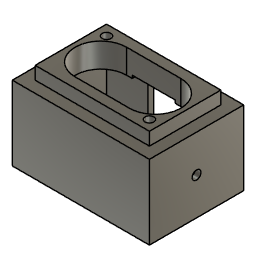
Chasy v39 (Autodesk Fusion 360 archive; units mm, degrees)
design "UltrasonicSensorSuport"
Autodesk Fusion 360 part; units mm, degrees
(part 1 of 2)
sketch "Base" plane through (0, 0, 0) normal (0, 0, 1) x (1, 0, 0) in component "UltrasonicSensorSuport"
  line L0 (18, 10.5) -> (-18, 10.5)
  line L1 (-18, 10.5) -> (-18, -10.5)
  line L2 (-18, -10.5) -> (18, -10.5)
  line L3 (18, -10.5) -> (18, 10.5)
  line L4 (18, 10.5) -> (-18, -10.5) construction
  line L5 (-18, 10.5) -> (18, -10.5) construction
  line L6 (-20, 12.5) -> (-20, -12.5)
  line L7 (-20, -12.5) -> (20, -12.5)
  line L8 (20, -12.5) -> (20, 12.5)
  line L9 (20, 12.5) -> (-20, 12.5)
  line L10 (-24, -16.5) -> (24, -16.5)
  line L11 (24, -16.5) -> (24, 16.5)
  line L12 (24, 16.5) -> (-24, 16.5)
  line L13 (-24, 16.5) -> (-24, -16.5)
  circle A0 centre (-16.4, 8.9) radius 1.55
  line L14 (0, 0) -> (-18, 0) construction
  line L15 (0, 0) -> (0, 10.5) construction
  circle A1 centre (-16.4, -8.9) radius 1.55
  circle A2 centre (16.4, 8.9) radius 1.55
  circle A3 centre (16.4, -8.9) radius 1.55
  line L16 (0, 10.5) -> (0, 12.5) construction
  line L17 (0, 12.5) -> (-5.5, 12.5) construction
  line L18 (-5.5, 7.5) -> (5.5, 7.5)
  line L19 (5.5, 7.5) -> (5.5, 19.5)
  line L20 (-5.5, 7.5) -> (-5.5, 19.5)
  line L21 (-5.5, 19.5) -> (5.5, 19.5)
  line L22 (0, 7.5) -> (0, 0) construction
  line L23 (5.5, 7.5) -> (8.5, 7.5) construction
  line L24 (8.5, 7.5) -> (8.5, 10.5) construction
  point P0 (0, 10.5)
  dimension "d8" = 36
  dimension "d9" = 21
  dimension "d12" = 2
  dimension "d13" = 6
  dimension "d46" = 3.1
  dimension "d47" = 1.6
  dimension "d48" = 1.6
  dimension "d52" = 11
  dimension "d53" = 12
  dimension "d54" = 3
  dimension "d55" = 3
  constraint horizontal L0
  constraint perpendicular L0 L1
  constraint parallel L0 L2
  constraint parallel L1 L3
  constraint coincident L4 L14.start
  constraint coincident L5 L14.start
  constraint coincident L14.start L15.start
  constraint midpoint L1 L14.end
  constraint midpoint L0 P0
  constraint symmetric A0 L14 A1
  constraint symmetric A0 L15 A2
  constraint symmetric L15 A1 A3
  constraint coincident P0 L15.end
  constraint midpoint L9 L16.end
  constraint coincident L9 L17.end
  constraint perpendicular L16 L17
  constraint perpendicular L15 L18
  constraint perpendicular L0 L19
  constraint perpendicular L12 L20
  constraint parallel L18 L21
  constraint midpoint L18 L22.start
  constraint perpendicular L18 L22
  constraint coincident L14.start L22
  constraint perpendicular L19 L23
  constraint coincident L0 L24.end
  constraint perpendicular L0 L24
  measures "d8" distance of L1.end L2.end
  measures "d9" distance of L0.end L1.end
  measures "d46" diameter of A0
  measures "d47" distance of L0 A0.centre
  measures "d48" distance of L1 A0.centre
  measures "d52" distance of L18.start L18.end
  measures "d53" distance of L18.end L19.end
  measures "d54" distance of L23.end L24.end
  measures "d55" distance of L18.end L23.end
extrude "Extrude1" add sketch "Base" along normal blind 3 contours L0 L1 L2 L3 L18 L19 L20 | L0 L1 L2 L3 L6 L7 L8 L9 L19 L20 | L0 L18 L19 L20 | L0 L9 L19 L20 | L6 L7 L8 L9 L10 L11 L12 L13 L19 L20 | L9 L12 L19 L20 | A0 | A1 | A2 | A3 makes body 1 in component "UltrasonicSensorSuport"
sketch "BaseExtension" plane through (0, 0, 3) normal (0, 0, 1) x (-1, 0, 0) in component "UltrasonicSensorSuport"
  line L0 (24, -16.5) -> (24, 16.5)
  line L1 (24, 16.5) -> (-24, 16.5)
  line L2 (-24, 16.5) -> (-24, -16.5)
  line L3 (-24, -16.5) -> (24, -16.5)
  line L4 (20, 12.5) -> (-20, 12.5)
  line L5 (-20, 12.5) -> (-20, -12.5)
  line L6 (-20, -12.5) -> (20, -12.5)
  line L7 (20, -12.5) -> (20, 12.5)
  circle A0 centre (-20.35, 12.85) radius 1.55
  circle A1 centre (20.35, -12.85) radius 1.55
  point P0 (-24, -16.5)
  point P1 (24, -16.5)
  point P2 (24, 16.5)
  point P3 (-24, 16.5)
  dimension "d16" = -4
  dimension "d19" = 3.1
  dimension "d20" = 3.1
  dimension "d21" = 3.65
  dimension "d22" = 3.65
  dimension "d23" = 3.65
  dimension "d24" = 3.65
  measures "d19" diameter of A0
  measures "d20" diameter of A1
  measures "d21" distance of L1 A0.centre
  measures "d22" distance of L2 A0.centre
  measures "d23" distance of L3 A1.centre
  measures "d24" distance of L0 A1.centre
extrude "Extrude2" add sketch "BaseExtension" along normal blind 6.5 separate body contours L4 L5 L6 L7 A0 A1 | L4 L5 A0 | L6 L7 A1 picked at (-19.557, 11.9554) picked at (19.557, -11.9554) makes body 2 in component "UltrasonicSensorSuport"
shell "Shell1" thickness 2 removed faces 1 at (1.8333, -5.5, 0) on bodies 1 in component "UltrasonicSensorSuport"
sketch "TransducerHoles" plane through (0, 0, 9.5) normal (0, 0, 1) x (-1, 0, 0) in component "UltrasonicSensorSuport"
  line L0 (20, -12.5) -> (20, 12.5)
  line L1 (20, 12.5) -> (-20, 12.5)
  line L2 (-20, 12.5) -> (-20, -12.5)
  line L3 (-20, -12.5) -> (20, -12.5)
  circle A0 centre (-9.5, 0) radius 9
  circle A1 centre (9.5, 0) radius 9
  line L4 (20, -12.5) -> (20, 12.5)
  line L5 (-20, 12.5) -> (-20, -12.5)
  line L6 (20, 0) -> (-20, 0) construction
  line L7 (24, -16.5) -> (24, 16.5)
  line L8 (-24, -16.5) -> (24, -16.5)
  line L9 (24, 16.5) -> (-24, 16.5)
  line L10 (-24, 16.5) -> (-24, -16.5)
  line L11 (-20, -12.5) -> (20, -12.5)
  line L12 (20, 12.5) -> (-20, 12.5)
  line L13 (0, -12.5) -> (0, 12.5) construction
  line L14 (9.5, 0) -> (0, 0) construction
  line L15 (0, 0) -> (-9.5, 0) construction
  line L16 (9.5, -9) -> (-9.5, -9)
  line L17 (9.5, 9) -> (-9.5, 9)
  dimension "d33" = 18
  dimension "d34" = 18
  dimension "d35" = 19
  constraint midpoint L4 L6.start
  constraint midpoint L5 L6.end
  constraint coincident A1.centre L6
  constraint coincident A0.centre L6
  constraint midpoint L11 L13.start
  constraint midpoint L12 L13.end
  constraint coincident A1.centre L14.start
  constraint coincident L14.end L15.start
  constraint perpendicular L13 L14
  constraint coincident A0.centre L15.end
  constraint perpendicular L13 L15
  constraint equal L14 L15
  constraint coincident A1 L16.start
  constraint coincident A0 L16.end
  constraint tangent A0 L16
  constraint tangent A1 L16
  constraint coincident A1 L17.start
  constraint coincident A0 L17.end
  constraint tangent A1 L17
  constraint tangent A0 L17
  measures "d33" diameter of A0
  measures "d34" diameter of A1
  measures "d35" distance of A0.centre A1.centre
extrude "Extrude7" cut sketch "TransducerHoles" against normal up to surface (9.5 mm away) contours A0 | A0 A1 L16 L17 | A1 bodies 1 2 in component "UltrasonicSensorSuport"
extrude "Extrude8" add 1 faces at (-3.1667, 14, 3) along direction (0, 0, 1) blind 2 on bodies 1 bodies 1 2 in component "UltrasonicSensorSuport"
extrude "Extrude9" cut sketch "Base" along normal up to surface (9.5 mm away) contours A0 | A3 bodies 1 in component "UltrasonicSensorSuport"
extrude "Extrude11" add 1 faces at (7.3333, -15.8333, 0) along direction (0, 0, -1) blind 21 on bodies 1 bodies 1 in component "UltrasonicSensorSuport"
extrude "Extrude10" cut sketch "Base" along normal blind 2 contours L0 L18 L19 L20 | L0 L9 L19 L20 | L9 L12 L19 L20 | L12 L19 L20 L21 bodies 1 in component "UltrasonicSensorSuport"
extrude "Extrude14" cut 1 faces at (-1.8333, 15.1667, 0) along direction (0, 0, -1) up to surface (21 mm away) on bodies 1 bodies 1 in component "UltrasonicSensorSuport"
extrude "Extrude16" cut 1 faces at (-5.5, 15.8333, -6) along direction (-1, 0, 0) blind 2 on bodies 1 bodies 1 in component "UltrasonicSensorSuport"
extrude "Extrude17" cut 1 faces at (5.5, 15.8333, -6) along direction (1, 0, 0) blind 2 on bodies 1 bodies 1 in component "UltrasonicSensorSuport"
sketch "MountingScrewHole" plane through (24, 0, 0) normal (1, 0, 0) x (0, 1, 0) in component "UltrasonicSensorSuport"
  line L0 (16.5, -21) -> (16.5, 5)
  line L1 (16.5, 5) -> (-16.5, 5)
  line L2 (-16.5, 5) -> (-16.5, -21)
  line L3 (16.5, 5) -> (-16.5, -21) construction
  line L4 (16.5, -21) -> (-16.5, 5) construction
  circle A0 centre (0, -8) radius 1.55
  line L5 (-16.5, -21) -> (16.5, -21)
  point P0 (0, -8)
  dimension "d63" = 3.1
  constraint coincident L0.end L1.start
  constraint coincident L2.end L3.end
  constraint coincident L0.start L4.start
  constraint coincident L1.end L2.start
  constraint midpoint L3 P0
  constraint coincident P0 A0.centre
  measures "d63" diameter of A0
extrude "Extrude13" cut sketch "MountingScrewHole" against normal up to surface (2 mm away) contours A0 bodies 1 in component "UltrasonicSensorSuport"
ref_plane "WorkPlane1" through (0, 0, -8) normal (1, 0, 0) x (0, 1, 0) in component "UltrasonicSensorSuport"
mirror "Mirror1" about plane through (0, 0, -8) normal (1, 0, 0) of "Extrude13" in component "UltrasonicSensorSuport"
pattern_linear "00000000-0000-0000-0000-000000000000" [suppressed]
component "UltrasonicSensorSuport" placed x (1, 0, 0) y (0, 1, 0) z (0, 0, 1) at (0, 0, 0)
equation "M3 = 3 mm"
equation "Length = 3.6 cm"
equation "Width = 2.1 cm"
equation "Height = 1 mm"
equation "TransducerHeight = 1.3 cm"
equation "TransducerDiameter = 1.6 cm"
equation "TransducersCenterDistance = 3.5 cm - TransducerDiameter"
equation "d8 = Length"
equation "d9 = Width"
equation "PrintMargin = 2 mm"
equation "BaseThickness = 3 mm"
equation "d12 = PrintMargin"
equation "d13 = PrintMargin + BaseThickness + 1 mm"
equation "d14 = BaseThickness"
equation "d16 = -PrintMargin - 2 mm"
equation "d17 = TransducerHeight / 2"
equation "d19 = M3 + 0.1 mm"
equation "d20 = d19"
equation "d21 = M3 / 2 + 0.15 mm + 2 mm"
equation "d22 = M3 / 2 + 0.15 mm + 2 mm"
equation "d23 = d22"
equation "d24 = d21"
equation "d33 = TransducerDiameter + PrintMargin"
equation "d34 = d33"
equation "d35 = TransducersCenterDistance"
equation "d37 = PrintMargin"
equation "d40 = PrintMargin"
equation "d46 = M3 + 0.1 mm"
equation "d47 = 0.1 mm + M3 / 2"
equation "d48 = d47"
equation "d63 = M3 + 0.1 mm"

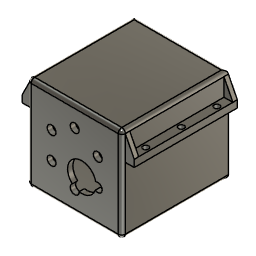
design "MotorEnclosure"
Autodesk Fusion 360 part; units mm, degrees
sketch "Front" plane through (0, 0, 0) normal (0, 1, 0) x (1, 0, 0)
  line L0 (23.5, -23.5) -> (-23.5, -23.5)
  line L1 (-23.5, -23.5) -> (-23.5, 23.5)
  line L2 (-23.5, 23.5) -> (23.5, 23.5)
  line L3 (23.5, 23.5) -> (23.5, -23.5)
  line L4 (23.5, -23.5) -> (-23.5, 23.5) construction
  line L5 (-23.5, -23.5) -> (23.5, 23.5) construction
  line L6 (-26.5, 26.5) -> (26.5, 26.5)
  line L7 (26.5, 26.5) -> (26.5, -26.5)
  line L8 (26.5, -26.5) -> (-26.5, -26.5)
  line L9 (-26.5, -26.5) -> (-26.5, 26.5)
  circle A0 centre (3.9904, -6.933) radius 8
  circle A1 centre (0, -15) radius 2.5
  circle A2 centre (12.9904, -7.5) radius 2.5
  circle A3 centre (12.9904, 7.5) radius 2.5
  circle A4 centre (0, 15) radius 2.5
  circle A5 centre (-12.9904, 7.5) radius 2.5
  circle A6 centre (-12.9904, -7.5) radius 2.5
  line L10 (0, 0) -> (0, -23.5) construction
  line L11 (-23.5, 0) -> (23.5, 0)
  circle A7 centre (3.9904, 6.933) radius 8
  dimension "d13" = 47
  dimension "d14" = 47
  dimension "d23" = 16
  dimension "d26" = 5
  dimension "d27" = 15
  dimension "d29" = 360
  dimension "d53" = 9
  dimension "d54" = 9
  constraint horizontal L0
  constraint perpendicular L0 L1
  constraint parallel L0 L2
  constraint parallel L1 L3
  constraint coincident L4 L10.start
  constraint coincident L5 L10.start
  constraint coincident L10.start origin
  constraint midpoint L0 L10.end
  constraint coincident A1.centre L10
  constraint midpoint L1 L11.start
  constraint midpoint L3 L11.end
  constraint symmetric A0 L11 A7
  measures "d13" distance of L1.end L2.end
  measures "d14" distance of L0.end L1.end
  measures "d23" diameter of A0
  measures "d26" diameter of A1
  measures "d27" vertical distance of L10.start A1.centre
  measures "d53" distance of A0.centre A1.centre
  measures "d54" horizontal distance of A0.centre A2.centre
extrude "Extrude4" add sketch "Front" along normal blind 3 contours L0 L1 L3 A0 A1 A2 L11 | L1 L2 L3 A3 A4 L11 A7 | A0 L11 | L11 A7 | A0 A1 A2 A7 | A0 A3 A4 A7 | A0 A2 | A0 A2 | A3 A7 | A3 A7 | A0 A1 | A0 A1 | A4 A7 | A4 A7 | A5 | A6 makes body 1
extrude "Extrude5" add sketch "Front" along normal blind 60 contours L6 L7 L8 L9 bodies 1
extrude "Extrude6" cut sketch "Front" along normal up to surface (3 mm away) contours A0 L11 | L11 A7 | A0 A3 A4 A7 | A3 A7 | A4 A7 picked at (11.4757, 7.3646) picked at (0.1211, 13.399) bodies 1
extrude "Extrude7" cut sketch "Front" along normal up to surface (3 mm away) contours A0 A2 | A0 A2 | A3 A7 | A3 A7 | A0 A1 | A0 A1 | A4 A7 | A4 A7 | A5 | A6 bodies 1
sketch "BottomHole" plane through (0, 0, -26.5) normal (0, 0, -1) x (1, 0, 0)
  line L0 (26.5, 0) -> (-26.5, 0)
  line L1 (-26.5, 0) -> (-26.5, -60)
  line L2 (-26.5, -60) -> (26.5, -60)
  line L3 (26.5, -60) -> (26.5, 0)
  line L4 (-23.5, -3) -> (23.5, -3)
  line L5 (23.5, -3) -> (23.5, -60)
  line L6 (23.5, -60) -> (-23.5, -60)
  line L7 (-23.5, -60) -> (-23.5, -3)
  line L8 (23.5, -3) -> (23.5, -33)
  line L9 (23.5, -33) -> (0, -25.5905)
  line L10 (0, -25.5905) -> (-23.5, -33)
  line L11 (-23.5, -33) -> (23.5, -33)
  line L12 (16.4289, -3) -> (23.5, -10.0711)
  line L13 (0, -3) -> (0, -25.5905)
  line L14 (-16.4289, -3) -> (-23.5, -10.0711)
  dimension "d55" = 30
  dimension "d57" = 145
  dimension "d60" = 45
  dimension "d61" = 5
  constraint coincident L4.end L5.start
  constraint perpendicular L4 L8
  constraint coincident L7 L10.end
  constraint perpendicular L8 L11
  constraint equal L9 L10
  constraint coincident L4 L12.start
  constraint coincident L8 L12.end
  constraint midpoint L4 L13.start
  constraint symmetric L12.start L13 L14.start
  constraint symmetric L12.end L13 L14.end
  measures "d55" distance of L4.end L8.end
  measures "d57" angle of L9 L10
  measures "d60" angle of L4 L12
  measures "d61" distance of L4.end L12
fillet "Fillet1" radius 2 6 edges at (26.5, 30, 26.5) (-26.5, 30, 26.5) (-26.5, 30, -26.5) (26.5, 30, -26.5) (0, 60, -26.5) (0, 60, 26.5) on bodies 1
fillet "Fillet2" radius 2 8 edges at (-25.9142, 0, 25.9142) (-26.5, 0, 0) (-25.9142, 0, -25.9142) (0, 0, -26.5) (25.9142, 0, -25.9142) (26.5, 0, 0) (25.9142, 0, 25.9142) (0, 0, 26.5) on bodies 1
sketch "Mounting" plane through (-26.5, 0, 0) normal (-1, 0, 0) x (0, -1, 0)
  line L0 (-2, -24.5) -> (-2, 24.5)
  line L1 (-2, 24.5) -> (-60, 24.5)
  line L2 (-60, 24.5) -> (-60, -24.5)
  line L3 (-60, -24.5) -> (-2, -24.5)
  line L4 (-60, 14.5) -> (-2, 14.5)
  line L5 (-2, 14.5) -> (-2, 10.5)
  line L6 (-2, 10.5) -> (-60, 10.5)
  line L7 (-60, 14.5) -> (-60, 10.5)
  dimension "d36" = 4
  dimension "d37" = 10
  constraint coincident L2 L4.start
  constraint coincident L0 L4.end
  constraint perpendicular L0 L4
  constraint coincident L0 L5.end
  constraint coincident L2 L6.end
  constraint perpendicular L2 L6
  measures "d36" distance of L4.end L5.end
  measures "d37" distance of L1 L4
extrude "Extrude8" add sketch "Mounting" along normal blind 5 separate body contours L0 L2 L4 L5 L6 L7 makes body 2
sketch "ScrewHoles" plane through (0, 0, 14.5) normal (0, 0, 1) x (-1, 0, 0)
  line L0 (26.5, -60) -> (31.5, -60)
  line L1 (31.5, -60) -> (31.5, -2)
  line L2 (31.5, -2) -> (26.5, -2)
  line L3 (26.5, -2) -> (24.5, -2)
  line L4 (24.5, -2) -> (24.5, -58)
  line L5 (26.5, -60) -> (24.5, -58)
  line L6 (26.5, -60) -> (26.5, -2)
  circle A0 centre (29, -51) radius 1.6
  circle A1 centre (29, -31) radius 1.6
  circle A2 centre (29, -11) radius 1.6
  line L7 (26.5, -60) -> (31.5, -2) construction
  line L8 (31.5, -60) -> (26.5, -2) construction
  line L9 (26.5, -2) -> (26.5, -60)
  dimension "d40" = 3.2
  dimension "d43" = 0
  dimension "d44" = 20
  constraint coincident L0.start L5.start
  constraint coincident L1.end L2.start
  constraint coincident A1.centre L7
  constraint coincident L0.end L1.start
  constraint coincident L2.end L3.start
  constraint coincident A1.centre L8
  measures "d40" diameter of A0
extrude "Extrude9" cut sketch "ScrewHoles" against normal up to surface (4 mm away) contours A0 | A1 | A2 bodies 1 2
sketch "Sketch5" plane through (0, 60, 0) normal (0, 1, 0) x (-1, 0, 0)
  line L0 (23.5, -23.5) -> (-23.5, -23.5)
  line L1 (-23.5, -23.5) -> (-23.5, 23.5)
  line L2 (-23.5, 23.5) -> (23.5, 23.5)
  line L3 (23.5, 23.5) -> (23.5, -23.5)
  line L4 (-26.5, -24.5) -> (26.5, -24.5)
  line L5 (26.5, -24.5) -> (26.5, 24.5)
  line L6 (26.5, 24.5) -> (-26.5, 24.5)
  line L7 (-26.5, 24.5) -> (-26.5, -24.5)
  line L8 (26.5, 14.5) -> (31.5, 14.5)
  line L9 (26.5, -24.5) -> (26.5, 24.5)
  line L10 (26.5, 24.5) -> (31.5, 14.5)
  constraint coincident L5.end L6.start
extrude "Extrude10" add sketch "Sketch5" against normal blind 2.5 separate body contours L5 L8 L9 L10 makes body 3
ref_plane "WorkPlane1" through (-29, 31, 12.5) normal (0, 1, 0) x (0, 0, -1)
mirror "Mirror1" about plane through (-29, 31, 12.5) normal (0, 1, 0) of bodies 3 makes body 4
combine "Combine1" operation add target body 2 tool bodies 3 4
mirror "Mirror2" about plane through (0, 0, 0) normal (1, 0, 0) of bodies 2 makes body 5
combine "Combine2" operation add target body 1 tool bodies 5 2
equation "Diameter = 37 mm"
equation "Length = 50 mm"
equation "ShaftDiameter = 6 mm"
equation "ShaftLength = 15 mm"
equation "PrintThickness = 3 mm"
equation "d13 = Diameter + 10 mm"
equation "d14 = d13"
equation "d18 = -PrintThickness"
equation "d19 = PrintThickness"
equation "d21 = Length + 10 mm"
equation "d23 = ShaftDiameter + 10 mm"

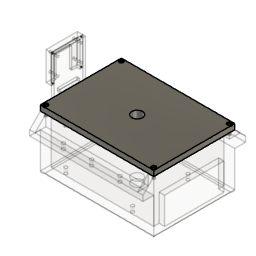
design "RasberryPiCase"
Autodesk Fusion 360 part; units mm, degrees
sketch "Base" plane through (0, 0, 0) normal (0, 0, 1) x (1, 0, 0) in component "Case"
  line L0 (42.5, 27.5) -> (-42.5, 27.5)
  line L1 (-42.5, 27.5) -> (-42.5, -27.5)
  line L2 (-42.5, -27.5) -> (42.5, -27.5)
  line L3 (42.5, -27.5) -> (42.5, 27.5)
  line L4 (42.5, 27.5) -> (-42.5, -27.5) construction
  line L5 (-42.5, 27.5) -> (42.5, -27.5) construction
  line L6 (-47.5, -32.5) -> (47.5, -32.5)
  line L7 (47.5, -32.5) -> (47.5, 32.5)
  line L8 (47.5, 32.5) -> (-47.5, 32.5)
  line L9 (-47.5, 32.5) -> (-47.5, -32.5)
  line L10 (-52.5, -37.5) -> (52.5, -37.5)
  line L11 (52.5, -37.5) -> (52.5, 37.5)
  line L12 (52.5, 37.5) -> (-52.5, 37.5)
  line L13 (-52.5, 37.5) -> (-52.5, -37.5)
  circle A0 centre (-40.7, -25.7) radius 1.5
  circle A1 centre (-40.7, 25.7) radius 1.5
  circle A2 centre (21, 25.7) radius 1.5
  circle A3 centre (21, -25.7) radius 1.5
  dimension "d6" = 85
  dimension "d7" = 55
  dimension "d9" = 5
  dimension "d10" = 10
  dimension "d12" = 3
  dimension "d13" = 3
  dimension "d14" = 3
  dimension "d15" = 3
  dimension "d22" = 1.8
  dimension "d23" = 1.8
  dimension "d24" = 1.8
  dimension "d25" = 1.8
  dimension "d26" = 1.8
  dimension "d27" = 1.8
  dimension "d28" = 21.5
  dimension "d29" = 21.5
  constraint horizontal L0
  constraint perpendicular L0 L1
  constraint parallel L0 L2
  constraint parallel L1 L3
  constraint coincident L4 origin
  constraint coincident L5 origin
  measures "d6" distance of L1.end L2.end
  measures "d7" distance of L0.end L1.end
  measures "d12" diameter of A0
  measures "d13" diameter of A1
  measures "d14" diameter of A2
  measures "d15" diameter of A3
  measures "d22" distance of L0 A1.centre
  measures "d23" distance of L1 A1.centre
  measures "d24" distance of L2 A0.centre
  measures "d25" distance of L2 A3.centre
  measures "d26" distance of L0 A2.centre
  measures "d27" distance of L1 A0.centre
  measures "d28" distance of L3 A2.centre
  measures "d29" distance of L3 A3.centre
extrude "Extrude1" add sketch "Base" along normal blind 50 contours L10 L11 L12 L13 makes body 1 in component "Case"
extrude "Extrude2" add sketch "Base" along normal blind 5 contours L0 L1 L2 L3 | L6 L7 L8 L9 bodies 1 in component "Case"
sketch "CableClearance" plane through (52.5, 0, 0) normal (1, 0, 0) x (0, 1, 0) in component "Case"
  line L0 (-37.5, 0) -> (37.5, 0)
  line L1 (37.5, 0) -> (37.5, 50)
  line L2 (37.5, 50) -> (-37.5, 50)
  line L3 (-37.5, 50) -> (-37.5, 0)
  line L4 (-27.5, 5) -> (-27.5, 30)
  line L5 (-27.5, 30) -> (27.5, 30)
  line L6 (27.5, 30) -> (27.5, 5)
  line L7 (-27.5, 30) -> (-37.5, 30) construction
  line L8 (27.5, 30) -> (37.5, 30) construction
  line L9 (-37.5, 0) -> (37.5, 0) construction
  line L10 (-27.2, 5) -> (-24.2, 5)
  line L11 (-27.2, 5) -> (-24.2, 5)
  line L12 (24.2, 5) -> (27.2, 5)
  line L13 (24.2, 5) -> (27.2, 5)
  line L14 (32.5, 5) -> (-32.5, 5)
  line L15 (-32.5, 5) -> (32.5, 5)
  dimension "d30" = 55
  dimension "d31" = 25
  constraint perpendicular L0 L4
  constraint perpendicular L4 L5
  constraint perpendicular L0 L6
  constraint coincident L3 L7.end
  constraint coincident L1 L8.end
  constraint parallel L8 L9
  constraint equal L7 L8
  constraint parallel L7 L9
  constraint coincident L6.end L14
  constraint coincident L4.start L15
  measures "d30" distance of L4.end L5.end
  measures "d31" distance of L4.start L4.end
extrude "Extrude3" cut sketch "CableClearance" against normal up to surface (5 mm away) contours L4 L5 L6 L10 L11 L12 L13 L14 L15 bodies 1 in component "Case"
fillet "Fillet1" radius 2 4 edges at (0, 37.5, 0) (52.5, 0, 0) (0, -37.5, 0) (-52.5, 0, 0) on bodies 1 in component "Case"
sketch "Sketch4" plane through (0, 0, 50) normal (0, 0, 1) x (-1, 0, 0) in component "Case"
  line L0 (47.5, 32.5) -> (47.5, -32.5)
  line L1 (47.5, -32.5) -> (-47.5, -32.5)
  line L2 (-47.5, -32.5) -> (-47.5, 32.5)
  line L3 (-47.5, 32.5) -> (47.5, 32.5)
  line L4 (52.5, -37.5) -> (52.5, 37.5)
  line L5 (52.5, 37.5) -> (-52.5, 37.5)
  line L6 (-52.5, 37.5) -> (-52.5, -37.5)
  line L7 (-52.5, -37.5) -> (52.5, -37.5)
  line L8 (52.5, -37.5) -> (47.5, -32.5) construction
  line L9 (47.5, -32.5) -> (52.5, -32.5) construction
  line L10 (47.5, -32.5) -> (47.5, -37.5) construction
  line L11 (52.5, -32.5) -> (47.5, -37.5) construction
  line L12 (52.5, 0) -> (0, 0) construction
  line L13 (0, 0) -> (0, -37.5) construction
  point P0 (57.5, 42.5)
  point P1 (50, -35)
  point P2 (50, 35)
  point P3 (-50, -35)
  point P4 (-50, 35)
  constraint coincident L4.start L7.end
  constraint coincident L0.end L1.start
  constraint coincident L4 L9.end
  constraint perpendicular L4 L9
  constraint coincident L7 L10.end
  constraint perpendicular L7 L10
  constraint midpoint L4 L12.start
  constraint coincident L12.end L13.start
  constraint midpoint L7 L13.end
  constraint midpoint L8 P1
  constraint symmetric L12 P1 P2
  constraint symmetric L13 P1 P3
  constraint symmetric L12 P3 P4
hole "Hole1" at (-50, 35, 50) at (50, 35, 50) at (-50, -35, 50) at (50, -35, 50) direction (0, 0, -1) diameter 2.529 depth 4 tip angle 118 bodies 1 in component "Case"
thread "Thread1" "ISO Metric profile 3.0 M3x0.5 6H" thread offset 0 thread depth 7.4 in component "Case"
sketch "Sketch1" plane through (0, 0, 50) normal (0, 0, 1) x (-1, 0, 0) in component "Lid"
  circle A0 centre (50, -35) radius 1.2645
  circle A1 centre (-50, -35) radius 1.2645
  circle A2 centre (50, 35) radius 1.2645
  line L0 (47.5, 32.5) -> (47.5, -32.5)
  line L1 (47.5, -32.5) -> (-47.5, -32.5)
  line L2 (-47.5, -32.5) -> (-47.5, 32.5)
  line L3 (-47.5, 32.5) -> (47.5, 32.5)
  line L4 (52.5, -37.5) -> (52.5, 37.5)
  line L5 (52.5, 37.5) -> (-52.5, 37.5)
  line L6 (-52.5, 37.5) -> (-52.5, -37.5)
  line L7 (-52.5, -37.5) -> (52.5, -37.5)
  circle A3 centre (-50, 35) radius 1.2645
extrude "Extrude1'" add sketch "Sketch1" along normal blind 5 separate body contours A0 | A1 | A2 | L0 L1 L2 L3 | L4 L5 L6 L7 | A3 makes body 2 in component "Lid"
extrude "Extrude2'" add sketch "Sketch1" against normal blind 2.5 contours L0 L1 L2 L3 bodies 2 in component "Lid"
sketch "Sketch2" plane through (0, 0, 55) normal (0, 0, 1) x (-1, 0, 0) in component "Lid"
  line L0 (-52.5, -37.5) -> (52.5, -37.5)
  line L1 (52.5, -37.5) -> (52.5, 37.5)
  line L2 (52.5, 37.5) -> (-52.5, 37.5)
  line L3 (-52.5, 37.5) -> (-52.5, -37.5)
  line L4 (52.5, 37.5) -> (-52.5, 37.5) construction
  line L5 (-52.5, 37.5) -> (-52.5, -37.5) construction
  line L6 (0, 37.5) -> (0, 0) construction
  line L7 (0, 0) -> (-52.5, 0) construction
  point P0 (-50, -35)
  point P1 (50, -35)
  point P2 (50, 35)
  point P3 (-50, 35)
  constraint midpoint L4 L6.start
  constraint coincident L6.end L7.start
  constraint midpoint L5 L7.end
  constraint symmetric P0 L7 P3
hole "Hole1'" at (-50, 35, 55) at (50, 35, 55) at (-50, -35, 55) at (50, -35, 55) direction (0, 0, -1) diameter 2.529 depth 10 tip angle 180 counterbore diameter 4 counterbore depth 1 bodies 2 in component "Lid"
thread "Thread1'" "ISO Metric profile 3.0 M3x0.5 6H" major diameter 3.086 minor diameter 2.529 pitch 0.5 angle 60 resizes the face on face at (50.8128, 35.9687, 52.6667) on face at (-49.1872, 35.9687, 52.6667) on face at (-49.1872, -34.0313, 52.6667) on face at (50.8128, -34.0313, 52.6667) on bodies 2 in component "Lid"
move_face "OffsetFaces2" offset -0.25 4 faces at (47.5, 10.8333, 48.3333) (15.8333, -32.5, 49.1667) (-47.5, -10.8333, 48.3333) (-15.8333, 32.5, 49.1667) on bodies 2 in component "Lid"
sketch "CameraBase" plane through (0, 0, 0) normal (0, 0, 1) x (1, 0, 0) in component "CameraModule v3"
  line L0 (12, 12) -> (-12, 12)
  line L1 (-12, 12) -> (-12, -12)
  line L2 (-12, -12) -> (12, -12)
  line L3 (12, -12) -> (12, 12)
  line L4 (12, 12) -> (-12, -12) construction
  line L5 (-12, 12) -> (12, -12) construction
  circle A0 centre (10.9, 10.9) radius 1.05
  line L6 (0, 0) -> (0, 12) construction
  circle A1 centre (10.9, -5) radius 1.05
  circle A2 centre (-10.9, -5) radius 1.05
  circle A3 centre (-10.9, 10.9) radius 1.05
  line L7 (-7.25, -12) -> (7.25, -12)
  line L8 (7.25, -12) -> (7.25, 8)
  line L9 (7.25, 8) -> (-7.25, 8)
  line L10 (-7.25, 8) -> (-7.25, -12)
  line L11 (-7.25, -2) -> (-12, -2) construction
  line L12 (7.25, -2) -> (12, -2) construction
  line L13 (14.5, -12) -> (14.5, 14.5)
  line L14 (14.5, 14.5) -> (-14.5, 14.5)
  line L15 (-14.5, 14.5) -> (-14.5, -12)
  line L16 (-14.5, -12) -> (-12, -12)
  line L17 (12, -12) -> (14.5, -12)
  dimension "d5" = 24
  dimension "d7_1" = 2.1
  dimension "d8" = 1.1
  dimension "d9_1" = 1.1
  dimension "d10_1" = 2.1
  dimension "d11" = 1.1
  dimension "d12_1" = 7
  dimension "d13_1" = 14.5
  dimension "d14_1" = 20
  dimension "d17_1" = 2.5
  constraint horizontal L0
  constraint perpendicular L0 L1
  constraint parallel L0 L2
  constraint parallel L1 L3
  constraint coincident L4 L6.start
  constraint coincident L5 L6.start
  constraint coincident L6.start origin
  constraint equal L0 L1
  constraint midpoint L0 L6.end
  constraint symmetric A0 L6 A3
  constraint symmetric L6 A1 A2
  constraint horizontal L7
  constraint vertical L8
  constraint horizontal L9
  constraint vertical L10
  constraint coincident L2 L7.start
  constraint midpoint L10 L11.start
  constraint coincident L1 L11.end
  constraint perpendicular L1 L11
  constraint midpoint L8 L12.start
  constraint coincident L3 L12.end
  constraint perpendicular L3 L12
  constraint equal L11 L12
  constraint perpendicular L1 L16
  constraint perpendicular L13 L17
  measures "d5" distance of L1.end L2.end
  measures "d7_1" diameter of A0
  measures "d8" distance of L3 A0.centre
  measures "d9_1" distance of L0 A0.centre
  measures "d10_1" diameter of A1
  measures "d11" distance of L3 A1.centre
  measures "d12_1" distance of L2 A1.centre
  measures "d13_1" distance of L7.start L7.end
  measures "d14_1" distance of L7.start L9.end
extrude "Extrude1''" add sketch "CameraBase" along normal blind 2 separate body contours L0 L1 L2 L3 L8 L9 L10 | L0 L1 L3 L13 L14 L15 L16 L17 makes body 3 in component "CameraModule v3"
extrude "Extrude2''" add sketch "CameraBase" against normal blind 3 contours L0 L1 L3 L13 L14 L15 L16 L17 bodies 3 in component "CameraModule v3"
sketch "CameraBaseEnclosure" plane through (0, 0, -3) normal (0, 0, -1) x (1, 0, 0) in component "CameraModule v3"
  line L0 (12, 12) -> (12, -12)
  line L1 (12, -12) -> (-12, -12)
  line L2 (-12, -12) -> (-12, 12)
  line L3 (-12, 12) -> (-14.5, 12)
  line L4 (-14.5, 12) -> (-14.5, -14.5)
  line L5 (-14.5, -14.5) -> (14.5, -14.5)
  line L6 (14.5, -14.5) -> (14.5, 12)
  line L7 (14.5, 12) -> (12, 12)
  circle A0 centre (10.9, -10.9) radius 1.05
  circle A1 centre (-10.9, -10.9) radius 1.05
  circle A2 centre (10.9, 5) radius 1.05
  circle A3 centre (-10.9, 5) radius 1.05
  line L8 (12, 12) -> (-12, 12)
  line L9 (-12.6726, -13.3274) -> (-12.9613, -12.8274)
  line L10 (-12.9613, -12.8274) -> (-13.5387, -12.8274)
  line L11 (-13.5387, -12.8274) -> (-13.8274, -13.3274)
  line L12 (-13.8274, -13.3274) -> (-13.5387, -13.8274)
  line L13 (-13.5387, -13.8274) -> (-12.9613, -13.8274)
  line L14 (-12.9613, -13.8274) -> (-12.6726, -13.3274)
  line L15 (-13.8274, -13.3274) -> (-14.5, -13.3274) construction
  line L16 (-12.6726, -13.3274) -> (-12, -13.3274) construction
  line L17 (-13.25, -13.8274) -> (-13.25, -14.5) construction
  line L18 (-12, -13.3274) -> (-12, -12) construction
  line L19 (-14.5, -1.25) -> (14.5, -1.25) construction
  line L20 (0, -1.25) -> (0, -14.5) construction
  line L21 (12.9613, -12.8274) -> (13.5387, -12.8274)
  line L22 (12.6726, -13.3274) -> (12.9613, -12.8274)
  line L23 (12.9613, -13.8274) -> (12.6726, -13.3274)
  line L24 (13.5387, -13.8274) -> (12.9613, -13.8274)
  line L25 (13.8274, -13.3274) -> (13.5387, -13.8274)
  line L26 (13.5387, -12.8274) -> (13.8274, -13.3274)
  line L27 (12.9613, 10.3274) -> (13.5387, 10.3274)
  line L28 (13.5387, 10.3274) -> (13.8274, 10.8274)
  line L29 (13.8274, 10.8274) -> (13.5387, 11.3274)
  line L30 (13.5387, 11.3274) -> (12.9613, 11.3274)
  line L31 (12.9613, 11.3274) -> (12.6726, 10.8274)
  line L32 (12.6726, 10.8274) -> (12.9613, 10.3274)
  line L33 (-12.6726, 10.8274) -> (-12.9613, 10.3274)
  line L34 (-12.9613, 11.3274) -> (-12.6726, 10.8274)
  line L35 (-13.5387, 11.3274) -> (-12.9613, 11.3274)
  line L36 (-13.8274, 10.8274) -> (-13.5387, 11.3274)
  line L37 (-13.5387, 10.3274) -> (-13.8274, 10.8274)
  line L38 (-12.9613, 10.3274) -> (-13.5387, 10.3274)
  point P0 (-13.25, -13.3274)
  point P1 (13.25, -13.3274)
  point P2 (13.25, 10.8274)
  point P3 (-13.25, 10.8274)
  dimension "d22_1" = 0.5
  constraint coincident L0.start L7.end
  constraint coincident L2.end L3.start
  constraint parallel L5 L10
  constraint coincident L4 L15.end
  constraint perpendicular L4 L15
  constraint coincident L2 L16.end
  constraint perpendicular L2 L16
  constraint midpoint L13 L17.start
  constraint coincident L5 L17.end
  constraint perpendicular L5 L17
  constraint equal L15 L17
  constraint equal L15 L16
  constraint coincident L1.end L2.start
  constraint midpoint L4 L19.start
  constraint midpoint L6 L19.end
  constraint midpoint L19 L20.start
  constraint midpoint L5 L20.end
  constraint symmetric L9.start L20 L22.start
  constraint symmetric L9.end L20 L21.start
  constraint symmetric L10.end L20 L21.end
  constraint symmetric L11.end L20 L25.start
  constraint symmetric L12.end L20 L24.start
  constraint symmetric L13.end L20 L23.start
  constraint symmetric P0 L20 P1
  constraint symmetric L9.start L19 L33.start
  constraint symmetric L9.end L19 L33.end
  constraint symmetric L10.end L19 L37.start
  constraint symmetric L11.end L19 L36.start
  constraint symmetric L12.end L19 L35.start
  constraint symmetric L13.end L19 L34.start
  constraint symmetric P0 L19 P3
  constraint symmetric L19 P1 P2
  constraint symmetric L19 L21.start L27.start
  constraint symmetric L19 L21.end L27.end
  constraint symmetric L19 L22.start L31.end
  constraint symmetric L19 L23.start L30.end
  constraint symmetric L19 L24.start L29.end
  constraint symmetric L19 L25.start L28.end
  measures "d22_1" distance of P0 L14
extrude "Extrude3'" add sketch "CameraBaseEnclosure" along normal blind 2.5 separate body contours L0 L1 L2 L3 L4 L5 L6 L7 | L0 L1 L2 L8 | L9 L10 L11 L12 L13 L14 | L21 L22 L23 L24 L25 L26 | L27 L28 L29 L30 L31 L32 | L33 L34 L35 L36 L37 L38 makes body 4 in component "CameraModule v3"
extrude "Extrude4" add sketch "CameraBaseEnclosure" against normal blind 0.25 contours L9 L10 L11 L12 L13 L14 | L21 L22 L23 L24 L25 L26 | L27 L28 L29 L30 L31 L32 | L33 L34 L35 L36 L37 L38 bodies 4 in component "CameraModule v3"
combine "Combine1" operation cut target body 3 tool bodies 4 keep tools in component "CameraModule v3"
extrude "Extrude5" add 1 faces at (4.8333, -12, -3.8333) along direction (0, -1, 0) blind 12.5 on bodies 4 bodies 4 in component "CameraModule v3"
sketch "Stand" plane through (0, 0, -5.5) normal (0, 0, -1) x (1, 0, 0) in component "CameraModule v3"
  circle A0 centre (-10.9, 5) radius 1.05
  circle A1 centre (10.9, 5) radius 1.05
  circle A2 centre (-10.9, -10.9) radius 1.05
  circle A3 centre (10.9, -10.9) radius 1.05
  line L0 (-14.5, 24.5) -> (-14.5, -14.5)
  line L1 (-14.5, -14.5) -> (14.5, -14.5)
  line L2 (14.5, -14.5) -> (14.5, 24.5)
  line L3 (14.5, 24.5) -> (-14.5, 24.5)
  line L4 (14.5, 24.5) -> (14.5, 21.5)
  line L5 (14.5, 21.5) -> (-14.5, 21.5)
  line L6 (-14.5, 21.5) -> (-14.5, 24.5)
  dimension "d28_1" = 3
  constraint coincident L2.end L3.start
  constraint perpendicular L3 L4
  constraint coincident L0 L5.end
  constraint perpendicular L0 L5
  constraint coincident L0.start L3.end
  measures "d28_1" distance of L2.end L4.end
extrude "Extrude6" add sketch "Stand" along normal blind 10 contours L0 L2 L3 L4 L5 L6 bodies 4 3 in component "CameraModule v3"
sketch "MountingHoles" plane through (0, -24.5, 0) normal (0, -1, 0) x (1, 0, 0) in component "CameraModule v3"
  line L0 (14.5, -3) -> (-14.5, -3)
  line L1 (-14.5, -3) -> (-14.5, -15.5)
  line L2 (-14.5, -15.5) -> (14.5, -15.5)
  line L3 (14.5, -15.5) -> (14.5, -3)
  line L4 (14.5, -9.25) -> (-14.5, -9.25) construction
  line L5 (0, -15.5) -> (0, -3) construction
  line L6 (14.5, -9.25) -> (0, -9.25) construction
  line L7 (7.25, -9.25) -> (7.25, -15.5) construction
  line L8 (7.25, -9.25) -> (7.25, -3) construction
  point P0 (-7.25, -9.25)
  constraint midpoint L3 L4.start
  constraint midpoint L1 L4.end
  constraint midpoint L2 L5.start
  constraint midpoint L0 L5.end
  constraint midpoint L4 L6.end
  constraint midpoint L6 L7.start
  constraint coincident L2 L7.end
  constraint perpendicular L2 L7
  constraint coincident L0 L8.end
  constraint perpendicular L0 L8
  constraint symmetric L5 L7.start P0
hole "Hole1''" at (7.25, -24.5, -9.25) at (-7.25, -24.5, -9.25) direction (0, 1, 0) diameter 3.05 end up to surface (3 mm away) bodies 3 4 in component "CameraModule v3"
sketch "ElectronicsHole" plane through (0, 0, -5.5) normal (0, 0, -1) x (1, 0, 0) in component "CameraModule v3"
  line L0 (14.5, 21.5) -> (-14.5, 21.5)
  line L1 (-14.5, 21.5) -> (-14.5, -14.5)
  line L2 (-14.5, -14.5) -> (14.5, -14.5)
  line L3 (14.5, -14.5) -> (14.5, 21.5)
  circle A0 centre (-10.9, 5) radius 1.05
  circle A1 centre (10.9, 5) radius 1.05
  circle A2 centre (-10.9, -10.9) radius 1.05
  circle A3 centre (10.9, -10.9) radius 1.05
  line L4 (9, 16.5) -> (-9, 16.5)
  line L5 (-9, 16.5) -> (-9, 19)
  line L6 (-9, 19) -> (9, 19)
  line L7 (9, 19) -> (9, 16.5)
  line L8 (9, 17.75) -> (14.5, 17.75) construction
  line L9 (-9, 17.75) -> (-14.5, 17.75) construction
  dimension "d33_1" = 18
  dimension "d34_1" = 2.5
  dimension "d35_1" = 2.5
  constraint horizontal L4
  constraint vertical L5
  constraint horizontal L6
  constraint vertical L7
  constraint midpoint L7 L8.start
  constraint coincident L3 L8.end
  constraint perpendicular L3 L8
  constraint midpoint L5 L9.start
  constraint coincident L1 L9.end
  constraint perpendicular L1 L9
  constraint equal L8 L9
  measures "d33_1" distance of L4.start L4.end
  measures "d34_1" distance of L4.start L6.end
  measures "d35_1" distance of L0 L6
extrude "Extrude7" cut sketch "ElectronicsHole" against normal up to surface (2.5 mm away) contours L4 L5 L6 L7 bodies 3 4 in component "CameraModule v3"
sketch "CameraMount" plane through (-52.5, 0, 0) normal (-1, 0, 0) x (0, -1, 0) in component "Case"
  line L0 (-37.5, 2) -> (37.5, 2)
  line L1 (37.5, 2) -> (37.5, 50)
  line L2 (37.5, 50) -> (-37.5, 50)
  line L3 (-37.5, 50) -> (-37.5, 2)
  line L4 (-15, 40) -> (15, 40)
  line L5 (15, 40) -> (15, 35)
  line L6 (15, 35) -> (-15, 35)
  line L7 (-15, 35) -> (-15, 40)
  line L8 (-15, 37.5) -> (-37.5, 37.5) construction
  line L9 (15, 37.5) -> (37.5, 37.5) construction
  dimension "d63" = 30
  dimension "d64" = 5
  constraint horizontal L4
  constraint vertical L5
  constraint horizontal L6
  constraint vertical L7
  constraint midpoint L7 L8.start
  constraint coincident L3 L8.end
  constraint perpendicular L3 L8
  constraint midpoint L5 L9.start
  constraint coincident L1 L9.end
  constraint perpendicular L1 L9
  constraint equal L8 L9
  measures "d63" distance of L4.start L4.end
  measures "d64" distance of L4.start L6.end
extrude "Extrude4'" add sketch "CameraMount" along normal blind 13 contours L4 L5 L6 L7 bodies 1 in component "Case"
sketch "MountingHoles (2)" plane through (0, 0, 40) normal (0, 0, 1) x (-1, 0, 0) in component "Case"
  line L0 (52.5, 15) -> (52.5, -15)
  line L1 (52.5, -15) -> (65.5, -15)
  line L2 (65.5, -15) -> (65.5, 15)
  line L3 (65.5, 15) -> (52.5, 15)
  line L4 (65.5, -14.5) -> (52.5, -14.5)
  line L5 (52.5, -14.5) -> (52.5, 14.5)
  line L6 (52.5, 14.5) -> (65.5, 14.5)
  line L7 (65.5, 14.5) -> (65.5, -14.5)
  line L8 (59, -14.5) -> (59, 14.5) construction
  line L9 (59, -14.5) -> (59, -15) construction
  line L10 (52.5, 0) -> (65.5, 0) construction
  line L11 (52.5, 0) -> (65.5, 14.5) construction
  line L12 (65.5, 0) -> (52.5, 14.5) construction
  point P0 (59, 7.25)
  point P1 (59, -7.25)
  dimension "d67" = 29
  dimension "d69" = 0.5
  constraint coincident L2 L4.start
  constraint coincident L0 L4.end
  constraint perpendicular L0 L4
  constraint coincident L0 L5.end
  constraint coincident L2 L6.end
  constraint perpendicular L2 L6
  constraint midpoint L4 L8.start
  constraint midpoint L6 L8.end
  constraint midpoint L1 L9.end
  constraint midpoint L5 L10.start
  constraint midpoint L2 L10.end
  constraint midpoint L12 P0
  constraint symmetric L10 P0 P1
  measures "d67" distance of L4.end L5.end
  measures "d69" distance of L8.start L9.end
hole "Hole2" at (-59, 7.25, 40) at (-59, -7.25, 40) direction (0, 0, -1) diameter 3.05 end up to surface (5 mm away) bodies 1 in component "Case"
sketch "SupportTriangle" plane through (0, -15, 0) normal (0, -1, 0) x (1, 0, 0) in component "Case"
  line L0 (-52.5, 35) -> (-52.5, 40)
  line L1 (-52.5, 40) -> (-65.5, 40)
  line L2 (-65.5, 40) -> (-65.5, 35)
  line L3 (-65.5, 35) -> (-52.5, 35)
  line L4 (-52.5, 2) -> (52.5, 2)
  line L5 (52.5, 2) -> (52.5, 50)
  line L6 (52.5, 50) -> (-52.5, 50)
  line L7 (-52.5, 50) -> (-52.5, 2)
  line L8 (-65.5, 35) -> (-52.5, 25.6726)
  dimension "d72" = 16
  constraint coincident L2.end L3.start
  constraint coincident L7 L8.end
  measures "d72" distance of L2.end L8.end
extrude "Extrude5'" add sketch "SupportTriangle" against normal blind 2.5 contours L3 L7 L8 bodies 1 in component "Case"
ref_plane "WorkPlane1" through (-59, 0, 32.8363) normal (0, -1, 0) x (0, 0, 1) in component "Case"
mirror "Mirror1" about plane through (-59, 0, 32.8363) normal (0, -1, 0) of "Extrude5'" in component "Case"
sketch "CameraElectronicsHole" plane through (-52.5, 0, 0) normal (-1, 0, 0) x (0, -1, 0) in component "Case"
  line L0 (-15, 25.6726) -> (-15, 40)
  line L1 (-15, 40) -> (15, 40)
  line L2 (15, 40) -> (15, 25.6726)
  line L3 (15, 25.6726) -> (12.5, 25.6726)
  line L4 (12.5, 25.6726) -> (12.5, 35)
  line L5 (12.5, 35) -> (-12.5, 35)
  line L6 (-12.5, 35) -> (-12.5, 25.6726)
  line L7 (-12.5, 25.6726) -> (-15, 25.6726)
  line L8 (-37.5, 2) -> (37.5, 2)
  line L9 (37.5, 2) -> (37.5, 50)
  line L10 (37.5, 50) -> (-37.5, 50)
  line L11 (-37.5, 50) -> (-37.5, 2)
  line L12 (-9, 48) -> (9, 48)
  line L13 (9, 45.5) -> (-9, 45.5)
  line L14 (9, 48) -> (9, 45.5)
  line L15 (-9, 45.5) -> (-9, 48)
extrude "Extrude6'" cut sketch "CameraElectronicsHole" against normal up to surface (5 mm away) contours L12 L13 L14 L15 bodies 1 in component "Case"
sketch "Sketch3" plane through (-47.25, 0, 0) normal (-1, 0, 0) x (0, -1, 0)
  line L0 (32.25, 50) -> (-32.25, 50)
  line L1 (-32.25, 50) -> (-32.25, 47.5)
  line L2 (-32.25, 47.5) -> (32.25, 47.5)
  line L3 (32.25, 47.5) -> (32.25, 50)
  line L4 (-9, 48) -> (9, 48)
  line L5 (9, 48) -> (9, 45.5)
  line L6 (-9, 45.5) -> (-9, 48)
  line L7 (9, 45.5) -> (-9, 45.5)
extrude "Extrude3''" cut sketch "Sketch3" against normal blind 5 contours L2 L5 L6 L7 | L2 L4 L5 L6 bodies 2 in component "Lid"
sketch "ChasyMounting" plane through (0, -37.5, 0) normal (0, -1, 0) x (1, 0, 0) in component "Case"
  line L0 (-52.5, 2) -> (52.5, 2)
  line L1 (52.5, 2) -> (52.5, 50)
  line L2 (52.5, 50) -> (-52.5, 50)
  line L3 (-52.5, 50) -> (-52.5, 2)
  line L4 (-52.5, 40) -> (-65.5, 40)
  line L5 (-52.5, 40) -> (-52.5, 35)
  line L6 (-52.5, 40) -> (52.5, 40)
  line L7 (-52.5, 35) -> (52.5, 35)
  line L8 (52.5, 40) -> (52.5, 35)
  dimension "d87" = 5
  constraint coincident L4.start L5.start
  constraint coincident L3 L5.end
  constraint coincident L1 L6.end
  constraint perpendicular L1 L6
  constraint coincident L1 L7.end
  constraint perpendicular L1 L7
  measures "d87" distance of L4.start L5.end
extrude "Extrude7'" add sketch "ChasyMounting" along normal blind 10 separate body contours L1 L3 L5 L6 L7 L8 makes body 5 in component "Case"
sketch "ChasyMountingSuport" plane through (-52.5, 0, 0) normal (-1, 0, 0) x (0, -1, 0) in component "Case"
  line L0 (-9, 45.5) -> (-9, 48)
  line L1 (-9, 48) -> (9, 48)
  line L2 (9, 48) -> (9, 45.5)
  line L3 (9, 45.5) -> (-9, 45.5)
  line L4 (-15, 25.6726) -> (-15, 40)
  line L5 (-15, 40) -> (15, 40)
  line L6 (15, 40) -> (15, 25.6726)
  line L7 (15, 25.6726) -> (12.5, 25.6726)
  line L8 (12.5, 25.6726) -> (12.5, 35)
  line L9 (12.5, 35) -> (-12.5, 35)
  line L10 (-12.5, 35) -> (-12.5, 25.6726)
  line L11 (-12.5, 25.6726) -> (-15, 25.6726)
  line L12 (-37.5, 2) -> (37.5, 2)
  line L13 (37.5, 2) -> (37.5, 50)
  line L14 (37.5, 50) -> (-37.5, 50)
  line L15 (-37.5, 50) -> (-37.5, 2)
  line L16 (37.5, 40) -> (47.5, 40)
  line L17 (37.5, 2) -> (37.5, 50)
  line L18 (37.5, 50) -> (47.5, 40)
  constraint coincident L13.end L14.start
  constraint coincident L16.end L18.end
extrude "Extrude8" add sketch "ChasyMountingSuport" against normal blind 5 separate body contours L13 L16 L17 L18 makes body 6 in component "Case"
ref_plane "WorkPlane2" through (0, 0, 26) normal (-1, 0, 0) x (0, -1, 0) in component "Case"
mirror "Mirror2" about plane through (0, 0, 26) normal (-1, 0, 0) of "Extrude8" makes body 7 in component "Case"
sketch "ChasyMountingHoles" plane through (0, 0, 40) normal (0, 0, 1) x (-1, 0, 0) in component "Case"
  line L0 (52.5, 47.5) -> (-52.5, 47.5)
  circle A0 centre (26.25, 42.5) radius 1.55
  circle A1 centre (0, 42.5) radius 1.55
  circle A2 centre (-26.25, 42.5) radius 1.55
  line L1 (47.5, 37.5) -> (47.5, 47.5) construction
  line L2 (-47.5, 37.5) -> (-47.5, 47.5) construction
  line L3 (47.5, 42.5) -> (-47.5, 42.5) construction
  line L4 (52.5, 37.5) -> (-52.5, 37.5) construction
  line L5 (52.5, 37.5) -> (-52.5, 37.5) construction
  line L6 (0, 42.5) -> (0, 37.5) construction
  line L7 (0, 47.5) -> (0, 42.5) construction
  line L8 (52.5, 37.5) -> (0, 47.5) construction
  line L9 (0, 47.5) -> (-52.5, 37.5) construction
  line L10 (-52.5, 37.5) -> (52.5, 37.5)
  line L11 (52.5, 37.5) -> (52.5, 47.5)
  line L12 (-52.5, 47.5) -> (-52.5, 37.5)
  dimension "d94" = 3.1
  dimension "d95" = 3.1
  dimension "d96" = 3.1
  constraint midpoint L1 L3.start
  constraint midpoint L2 L3.end
  constraint coincident A0.centre L3
  constraint coincident A1.centre L3
  constraint coincident A2.centre L3
  constraint midpoint L3 A1.centre
  constraint midpoint L5 L6.end
  constraint coincident A1.centre L6
  constraint midpoint L0 L7.start
  constraint coincident A1.centre L6.start
  constraint coincident L4.start L5.start
  constraint coincident L4.end L5.end
  constraint coincident A2.centre L9
  constraint coincident A0.centre L8
  measures "d94" diameter of A0
  measures "d95" diameter of A1
  measures "d96" diameter of A2
extrude "Extrude9" cut sketch "ChasyMountingHoles" against normal up to surface (5 mm away) contours A0 | A1 | A2 bodies 5 6 1 in component "Case"
combine "Combine1'" operation add target body 5 tool bodies 6 7 in component "Case"
ref_plane "WorkPlane3" through (0, 0, 26) normal (0, -1, 0) x (1, 0, 0) in component "Case"
mirror "Mirror3" about plane through (0, 0, 26) normal (0, -1, 0) of bodies 5 makes body 8 in component "Case"
combine "Combine2" operation add target body 1 tool bodies 5 8 in component "Case"
hole "Hole3" at (0.1032, -0.4666, 0) direction (0, 0, 1) diameter 10 end up to surface (55 mm away) bodies 1 in component "Case"
hole "Hole2'" at (0.1032, -0.4666, 55) direction (0, 0, -1) diameter 10 end up to surface (50 mm away) bodies 2 in component "Lid"
component "Case" placed x (1, 0, 0) y (0, 1, 0) z (0, 0, 1) at (0, 0, 0)
component "Lid" placed x (1, 0, 0) y (0, 1, 0) z (0, 0, 1) at (0, 0, 0)
component "CameraModule v3" placed x (0, -1, 0) y (0, 0, 1) z (-1, 0, 0) at (-68.25, 0, 64.5)
equation "RasberryPiLength = 8.5 cm"
equation "RasberryPiWidth = 5.5 cm"
equation "RasberryPiHeight = 1.5 cm"
equation "CoolingClearance = 0.5 cm"
equation "TopClearance = 2 cm"
equation "d6 = RasberryPiLength"
equation "d7 = RasberryPiWidth"
equation "PrintThickness = 1 cm"
equation "d9 = CoolingClearance"
equation "d10 = PrintThickness"
equation "M2o5 = 3 mm"
equation "d12 = M2o5"
equation "d13 = M2o5"
equation "d14 = M2o5"
equation "d15 = M2o5"
equation "d16 = PrintThickness + RasberryPiHeight + TopClearance + CoolingClearance"
equation "d18 = PrintThickness / 2"
equation "d22 = ( 0.6 mm + M2o5 ) / 2"
equation "d23 = ( 0.6 mm + M2o5 ) / 2"
equation "d24 = d22"
equation "d25 = d22"
equation "d26 = d22"
equation "d27 = d23"
equation "d28 = 2.3 cm - M2o5 / 2"
equation "d29 = d28"
equation "d30 = RasberryPiWidth"
equation "d31 = RasberryPiHeight + 1 cm"
equation "d42 = PrintThickness / 2"
equation "d44 = -PrintThickness / 4"
equation "length = 24 mm"
equation "height = 6 mm"
equation "M2 = 2 mm"
equation "M3 = 3 mm"
equation "length_1 = 24 mm"
equation "height_1 = 6 mm"
equation "M2_1 = 2 mm"
equation "M3_1 = 3 mm"
equation "d5 = length_1"
equation "d7_1 = M2_1 + 0.1 mm"
equation "d10_1 = M2_1 + 0.1 mm"
equation "d11 = d8"
equation "d94 = M3 + 0.1 mm"
equation "d95 = d94"
equation "d96 = d94"

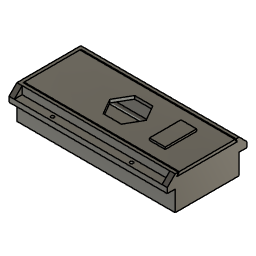
design "BatteryCase"
Autodesk Fusion 360 part; units mm, degrees
sketch "Base" plane through (0, 0, 0) normal (0, 0, 1) x (1, 0, 0)
  line L0 (72.5, 27.5) -> (-72.5, 27.5)
  line L1 (-72.5, 27.5) -> (-72.5, -27.5)
  line L2 (-72.5, -27.5) -> (72.5, -27.5)
  line L3 (72.5, -27.5) -> (72.5, 27.5)
  line L4 (72.5, 27.5) -> (-72.5, -27.5) construction
  line L5 (-72.5, 27.5) -> (72.5, -27.5) construction
  line L6 (-75.5, -30.5) -> (75.5, -30.5)
  line L7 (75.5, -30.5) -> (75.5, 30.5)
  line L8 (75.5, 30.5) -> (-75.5, 30.5)
  line L9 (-75.5, 30.5) -> (-75.5, -30.5)
  dimension "d5" = 145
  dimension "d6" = 55
  dimension "d7" = 3
  constraint horizontal L0
  constraint perpendicular L0 L1
  constraint parallel L0 L2
  constraint parallel L1 L3
  constraint coincident L4 origin
  constraint coincident L5 origin
  measures "d5" distance of L1.end L2.end
  measures "d6" distance of L0.end L1.end
extrude "Extrude1" add sketch "Base" along normal blind 3 contours L0 L1 L2 L3 | L6 L7 L8 L9 makes body 1
extrude "Extrude2" add sketch "Base" along normal blind 32 bodies 1
fillet "Fillet1" radius 2.5 8 edges at (0, 27.5, 3) (-72.5, 27.5, 17.5) (-72.5, 0, 3) (72.5, 0, 3) (72.5, 27.5, 17.5) (72.5, -27.5, 17.5) (-72.5, -27.5, 17.5) (0, -27.5, 3) on bodies 1
sketch "Cable Holes" plane through (-75.5, 0, 0) normal (-1, 0, 0) x (0, -1, 0)
  line L0 (-30.5, 0) -> (30.5, 0)
  line L1 (30.5, 0) -> (30.5, 32)
  line L2 (30.5, 32) -> (-30.5, 32)
  line L3 (-30.5, 32) -> (-30.5, 0)
  line L4 (-15, 0) -> (-15, 7.5) construction
  line L5 (-15, 7.5) -> (-15, 19.5)
  line L6 (-15, 19.5) -> (15, 19.5)
  line L7 (-15, 7.5) -> (15, 7.5)
  line L8 (15, 7.5) -> (15, 19.5)
  line L9 (15, 13.5) -> (30.5, 13.5) construction
  line L10 (-15, 13.5) -> (-30.5, 13.5) construction
  dimension "d14" = 7.5
  dimension "d15" = 12
  dimension "d16" = 30
  constraint coincident L0 L4.start
  constraint perpendicular L0 L4
  constraint perpendicular L2 L5
  constraint perpendicular L5 L6
  constraint perpendicular L4 L7
  constraint midpoint L8 L9.start
  constraint coincident L1 L9.end
  constraint perpendicular L1 L9
  constraint midpoint L5 L10.start
  constraint coincident L3 L10.end
  constraint perpendicular L3 L10
  constraint equal L9 L10
  constraint perpendicular L6 L8
  measures "d14" distance of L4.start L4.end
  measures "d15" distance of L4.end L5.end
  measures "d16" distance of L5.end L6.end
extrude "Extrude3" cut sketch "Cable Holes" against normal up to surface (3 mm away) contours L5 L6 L7 L8 bodies 1